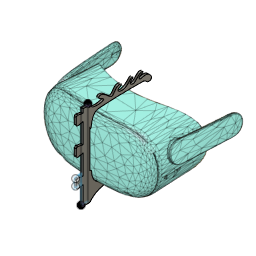
Quest Flat Holder To Store v1 (Autodesk Fusion 360 design; units mm, degrees)
Autodesk Fusion 360 part; units mm, degrees
other "Fonction de maillage de base1"
other "Modifier1"
sketch "Esquisse2" plane through (0, 0, 0) normal (1, 0, 0) x (0, 1, 0)
  line L0 (0, 0) -> (85, 0) construction
  line L1 (85, 0) -> (85, -20) construction
  line L2 (85, -20) -> (0, -20) construction
  line L3 (0, -20) -> (0, 0) construction
  spline S0 degree 5 poles (0, 20) (0.1728, 20.096) (0.5018, 20.2595) (0.9458, 20.4196) (1.4388, 20.4623) (1.8937, 20.2348) (2.1997, 19.7392) (2.3839, 19.0043) (2.486, 18.0734) (2.5511, 16.9974) (2.6227, 15.8294) (2.7376, 14.6194) (2.9173, 13.4073) (3.1676, 12.2219) (3.4842, 11.0828) (3.8558, 10.002) (4.2682, 8.9856) (4.7086, 8.0352) (5.1695, 7.1497) (5.6506, 6.3263) (6.1549, 5.5614) (6.688, 4.851) (7.2552, 4.1918) (7.8594, 3.582) (8.5004, 3.0212) (9.177, 2.5098) (9.8879, 2.0486) (10.6332, 1.6379) (11.416, 1.2771) (12.2414, 0.9646) (13.1157, 0.6985) (14.0453, 0.4767) (15.0358, 0.297) (16.0906, 0.1581) (17.2121, 0.0586) (18.4011, -0.0021) (19.4067, -0.0202) (20.1915, -0.0167) (20.7282, -0.0068) (21, 0) knots 0 0 0 0 0 0 0.028571 0.057143 0.085714 0.114286 0.142857 0.171429 0.2 0.228571 0.257143 0.285714 0.314286 0.342857 0.371429 0.4 0.428571 0.457143 0.485714 0.514286 0.542857 0.571429 0.6 0.628571 0.657143 0.685714 0.714286 0.742857 0.771429 0.8 0.828571 0.857143 0.885714 0.914286 0.942857 0.971429 1 1 1 1 1 1
  spline S1 degree 5 poles (0, -20) (0.5064, -19.2983) (1.5674, -17.9422) (3.3034, -16.0502) (5.9091, -13.8142) (9.6604, -11.5007) (13.9117, -9.6603) (18.656, -8.2562) (23.8646, -7.2118) (29.4972, -6.4287) (35.5074, -5.8004) (41.8485, -5.2261) (48.4776, -4.6251) (55.3593, -3.9458) (62.4652, -3.1575) (69.7745, -2.245) (75.7737, -1.4114) (80.3552, -0.7281) (83.4457, -0.247) (85, 0) knots 0 0 0 0 0 0 0.066667 0.133333 0.2 0.266667 0.333333 0.4 0.466667 0.533333 0.6 0.666667 0.733333 0.8 0.866667 0.933333 1 1 1 1 1 1
  spline S2 degree 5 poles (85, 0) (85.575, 0.0875) (86.7285, 0.3082) (88.4686, 0.7768) (90.8086, 1.677) (93.7558, 3.2561) (96.6909, 5.2678) (99.5457, 7.6663) (102.2047, 10.3705) (104.4963, 13.2564) (106.1711, 16.1422) (106.9676, 18.8127) (106.7051, 21.0543) (105.3645, 22.6857) (103.1826, 23.5917) (100.722, 23.753) (98.6234, 23.2199) (97.4016, 22.0921) (97.1788, 20.4954) (97.593, 18.5638) (98.0858, 16.4294) (98.097, 14.2122) (97.3281, 12.0076) (95.7145, 9.8887) (93.3441, 7.9095) (90.3947, 6.1092) (87.0665, 4.5151) (83.512, 3.1458) (79.8386, 2.0134) (76.1175, 1.1247) (72.3914, 0.4826) (69.4234, 0.1665) (67.2077, 0.0403) (65.7351, 0.0052) (65, 0) knots 0 0 0 0 0 0 0.033333 0.066667 0.1 0.133333 0.166667 0.2 0.233333 0.266667 0.3 0.333333 0.366667 0.4 0.433333 0.466667 0.5 0.533333 0.566667 0.6 0.633333 0.666667 0.7 0.733333 0.766667 0.8 0.833333 0.866667 0.9 0.933333 0.966667 1 1 1 1 1 1
  line L4 (0, 0) -> (0, 20)
  line L5 (21, 0) -> (65, 0)
  line L6 (0, 0) -> (0, -20)
  point P0 (2, 20)
  point P1 (2.6822, 15.27)
  point P2 (4.5, 8.5)
  point P3 (7, 4.5)
  point P4 (10, 2)
  point P5 (14, 0.5)
  point P6 (13.4129, -10)
  point P7 (40.3283, -5.3657)
  point P8 (102.6529, 11.0428)
  point P9 (105.3058, 22.3913)
  point P10 (97.9366, 22.3913)
  point P11 (98, 16)
  point P12 (90, 6)
  dimension "d3" = 85
  dimension "d4" = 20
  constraint horizontal L0
  constraint vertical L1
  constraint horizontal L2
  constraint vertical L3
  constraint coincident L0.start L3.end
  constraint coincident L0 S0.end
  constraint coincident L0 S2.end
  constraint perpendicular L0 L4
  measures "d3" distance of L0.start L0.end
  measures "d4" distance of L0.start L2.end
extrude "Extrusion1" add sketch "Esquisse2" along normal blind 3 makes body 1
sketch "Esquisse3" plane through (0, 0, 0) normal (1, 0, 0) x (0, 1, 0)
  line L0 (0, 94.6179) -> (85, 94.6179) construction
  line L1 (85, 94.6179) -> (85, 114.6179) construction
  line L2 (85, 114.6179) -> (0, 114.6179) construction
  line L3 (0, 114.6179) -> (0, 94.6179) construction
  line L4 (0, 94.6179) -> (0, 75)
  spline S0 degree 5 poles (2, 75) (2.0202, 75.3852) (2.0715, 76.1534) (2.1807, 77.2986) (2.3912, 78.8117) (2.7621, 80.6771) (3.2396, 82.5084) (3.8209, 84.2894) (4.5015, 85.9934) (5.2735, 87.579) (6.1296, 88.9972) (7.0689, 90.2031) (8.1023, 91.166) (9.258, 91.8812) (10.5862, 92.3785) (12.1486, 92.7086) (14.0103, 92.9314) (16.2308, 93.1038) (18.8544, 93.2665) (21.9061, 93.4406) (25.3926, 93.633) (29.3013, 93.8393) (33.6009, 94.0477) (38.24, 94.2424) (43.1479, 94.4068) (48.2328, 94.5281) (53.3833, 94.5985) (58.4639, 94.6234) (63.3238, 94.6152) (67.7739, 94.6186) (71.6525, 94.6526) (74.8757, 94.68) (77.4148, 94.6435) (79.3006, 94.4768) (80.6174, 94.1256) (81.5018, 93.5651) (82.137, 92.8177) (82.7573, 91.9753) (83.5789, 91.1727) (84.729, 90.5551) (86.1523, 90.2442) (87.6474, 90.3207) (88.9663, 90.8167) (89.8915, 91.7056) (90.3307, 92.8885) (90.2941, 94.2263) (89.8594, 95.5735) (89.1393, 96.8178) (88.2552, 97.8964) (87.3226, 98.7772) (86.4355, 99.4496) (85.8043, 99.8181) (85.3821, 99.9986) (85.1236, 100.0764) (85, 100.1046) knots 0 0 0 0 0 0 0.02 0.04 0.06 0.08 0.1 0.12 0.14 0.16 0.18 0.2 0.22 0.24 0.26 0.28 0.3 0.32 0.34 0.36 0.38 0.4 0.42 0.44 0.46 0.48 0.5 0.52 0.54 0.56 0.58 0.6 0.62 0.64 0.66 0.68 0.7 0.72 0.74 0.76 0.78 0.8 0.82 0.84 0.86 0.88 0.9 0.92 0.94 0.96 0.98 1 1 1 1 1 1
  line L5 (50.046, 94.6179) -> (76, 94.6179)
  spline S1 degree 5 poles (0, 75) (0.04, 74.8483) (0.12, 74.5582) (0.24, 74.1627) (0.4, 73.7162) (0.6, 73.3019) (0.8, 73.0442) (1, 72.956) (1.2, 73.0442) (1.4, 73.3019) (1.6, 73.7162) (1.76, 74.1627) (1.88, 74.5582) (1.96, 74.8483) (2, 75) knots 0 0 0 0 0 0 0.1 0.2 0.3 0.4 0.5 0.6 0.7 0.8 0.9 1 1 1 1 1 1
  line L6 (0, 94.6179) -> (0, 110)
  spline S2 degree 5 poles (0, 103.8612) (0.0594, 103.6458) (0.2491, 103.0393) (0.6491, 102.1073) (1.4026, 100.9699) (2.7032, 99.7974) (4.5145, 98.8515) (6.6398, 98.2367) (8.9921, 97.9297) (11.4551, 97.8986) (13.8795, 98.1029) (16.1006, 98.4961) (17.9568, 99.0296) (19.3078, 99.6559) (20.0524, 100.3325) (20.147, 101.025) (19.6236, 101.7106) (18.6074, 102.3817) (17.2834, 103.0411) (15.8653, 103.6979) (14.5626, 104.3634) (13.5514, 105.0463) (12.9359, 105.749) (12.7503, 106.4616) (12.9835, 107.155) (13.5974, 107.7726) (14.5449, 108.2285) (15.7707, 108.4296) (17.2154, 108.2956) (18.8182, 107.7781) (20.5203, 106.8841) (22.2667, 105.6788) (24.0079, 104.2665) (25.7004, 102.7783) (27.3086, 101.3566) (28.8054, 100.1412) (30.1742, 99.2545) (31.4094, 98.7879) (32.5181, 98.7853) (33.5207, 99.2355) (34.4477, 100.085) (35.3379, 101.2458) (36.2356, 102.6055) (37.1892, 104.0369) (38.2469, 105.4075) (39.4424, 106.5917) (40.782, 107.4827) (42.2327, 108.0039) (43.7068, 108.122) (45.054, 107.8564) (46.0348, 107.2969) (46.4036, 106.5721) (46.0116, 105.8057) (44.9262, 105.07) (43.4777, 104.3604) (42.1029, 103.6356) (41.1858, 102.8524) (40.98, 101.9881) (41.3072, 101.1045) (41.8959, 100.2884) (42.7, 99.5867) (43.7084, 99.0408) (44.9511, 98.6814) (46.4159, 98.543) (48.0582, 98.6571) (49.8113, 99.0469) (51.5976, 99.7212) (53.3396, 100.6684) (54.9707, 101.8501) (56.4453, 103.1961) (57.753, 104.5956) (58.9108, 105.9106) (59.9459, 107.0023) (60.8814, 107.752) (61.7197, 108.0872) (62.4307, 107.9988) (62.9269, 107.5773) (63.0956, 106.978) (62.8745, 106.3345) (62.3108, 105.6926) (61.5214, 105.0471) (60.6581, 104.3739) (59.8672, 103.6713) (59.2651, 102.9698) (58.9433, 102.2883) (58.9681, 101.5986) (59.3795, 100.7877) (60.1369, 99.9443) (61.1612, 99.226) (62.3546, 98.8155) (63.6313, 98.8337) (64.9349, 99.3) (66.2302, 100.1631) (67.5002, 101.3194) (68.7406, 102.6368) (69.9563, 103.9754) (71.156, 105.2098) (72.3483, 106.2513) (73.5347, 107.045) (74.7026, 107.5654) (75.8178, 107.8129) (76.8197, 107.8097) (77.6089, 107.5967) (78.0566, 107.227) (78.0583, 106.7528) (77.5908, 106.211) (76.7239, 105.6208) (75.589, 104.9939) (74.3615, 104.3412) (73.2363, 103.681) (72.4025, 103.0412) (71.97, 102.424) (71.9613, 101.8181) (72.1553, 101.104) (72.4975, 100.3787) (73.0531, 99.8457) (73.89, 99.6554) (75.0119, 99.7998) (76.3766, 100.1751) (77.9071, 100.6231) (79.5054, 100.9824) (81.0644, 101.1308) (82.4822, 101.0442) (83.6696, 100.7811) (84.378, 100.5037) (84.7522, 100.2982) (84.9294, 100.168) (85, 100.1046) knots 0.01975659 0.01975659 0.01975659 0.01975659 0.01975659 0.01975659 0.024 0.032 0.04 0.048 0.056 0.064 0.072 0.08 0.088 0.096 0.104 0.112 0.12 0.128 0.136 0.144 0.152 0.16 0.168 0.176 0.184 0.192 0.2 0.208 0.216 0.224 0.232 0.24 0.248 0.256 0.264 0.272 0.28 0.288 0.296 0.304 0.312 0.32 0.328 0.336 0.344 0.352 0.36 0.368 0.376 0.384 0.392 0.4 0.408 0.416 0.424 0.432 0.44 0.448 0.456 0.464 0.472 0.48 0.488 0.496 0.504 0.512 0.52 0.528 0.536 0.544 0.552 0.56 0.568 0.576 0.584 0.592 0.6 0.608 0.616 0.624 0.632 0.64 0.648 0.656 0.664 0.672 0.68 0.688 0.696 0.704 0.712 0.72 0.728 0.736 0.744 0.752 0.76 0.768 0.776 0.784 0.792 0.8 0.808 0.816 0.824 0.832 0.84 0.848 0.856 0.864 0.872 0.88 0.888 0.896 0.904 0.912 0.92 0.928 0.936 0.944 0.952 0.96 0.968 0.976 0.984 0.992 1 1 1 1 1 1
  line L7 (-2.2438, 111.9912) -> (2.2438, 95.7313)
  line L8 (41.0002, 107.9903) -> (41.2219, 96.0623)
  line L9 (59, 107.9346) -> (59, 96.0654)
  line L10 (72, 108.1104) -> (72, 95.8896)
  line L11 (82.3506, 102.4836) -> (87.6494, 97.7257)
  point P0 (4.0472, 84.8089)
  point P1 (8, 91)
  point P2 (15, 93)
  point P3 (63.023, 94.6179)
  point P4 (81.5564, 93.4173)
  point P5 (84, 91)
  point P6 (89, 91)
  point P7 (90, 95)
  point P8 (87, 99)
  point P9 (1, 73)
  point P10 (9, 98)
  point P11 (20, 101)
  point P12 (14.2323, 104.6179)
  point P13 (13, 107)
  point P14 (18, 108)
  point P15 (31, 99)
  point P16 (36.0384, 102.3089)
  point P17 (44, 108)
  point P18 (46, 106)
  point P19 (41.111, 102.0263)
  point P20 (44, 99)
  point P21 (55.43, 102.3089)
  point P22 (62, 108)
  point P23 (63, 107)
  point P24 (60.9799, 104.6179)
  point P25 (59, 102)
  point P26 (62, 99)
  point P27 (70, 104)
  point P28 (76.5063, 107.7784)
  point P29 (78, 107)
  point P30 (74.8889, 104.6179)
  point P31 (72, 102)
  point P32 (73, 100)
  point P33 (80, 101)
  dimension "d7" = 85
  dimension "d8" = 20
  constraint horizontal L0
  constraint vertical L1
  constraint horizontal L2
  constraint vertical L3
  constraint perpendicular L0 L4
  constraint coincident L0 P3
  constraint coincident L1 S0.end
  constraint midpoint P3 L5
  constraint coincident L0 L5.end
  constraint coincident L3 L6.end
  constraint coincident L3 S2.start
  constraint midpoint S2.start L7
  constraint midpoint P19 L8
  constraint midpoint P25 L9
  constraint midpoint P31 L10
  constraint midpoint S0.end L11
  measures "d7" distance of L0.start L0.end
  measures "d8" distance of L0.start L2.end
sketch "Esquisse4" plane through (0, 0, 0) normal (1, 0, 0) x (0, 1, 0)
  line L0 (0, 103.8612) -> (-10, 103.8612)
  line L1 (-10, 103.8612) -> (-10, -20)
  line L2 (-10, -20) -> (0, -20)
  line L3 (0, -20) -> (0, 103.8612)
  point P0 (0, 103.8612)
  dimension "d11" = 10
  constraint horizontal L0
  constraint vertical L1
  constraint horizontal L2
  constraint vertical L3
  constraint coincident P0 L0.start
  measures "d11" distance of P0 L0.end
extrude "Extrusion2" add sketch "Esquisse3" sketch "Esquisse4" along normal blind 3 contours L4 S0 S1 L6 S2 L8 L9 L10 | S2 L8 | S2 L9 | S2 L10 of sketch 2 bodies 1
sketch "Esquisse5" plane through (0, 0, 0) normal (1, 0, 0) x (0, 1, 0)
  line L0 (-10, -20) -> (-10, 20)
  line L1 (-10, 20) -> (-20, 20)
  line L2 (-20, 17.5851) -> (-20, 7.9635)
  line L3 (-20, 5.5) -> (-10, 5.5)
  line L4 (-10, 5.5) -> (-10, 20)
  line L5 (-17.6274, 19.5501) -> (-10, 18.1039)
  line L6 (-17.5891, 6.0061) -> (-10, 7.5994)
  arc A0 (-17.6274, 19.5501) -> (-20, 17.5851) centre (-18, 17.5851) ccw
  arc A1 (-20, 7.9635) -> (-17.5891, 6.0061) centre (-18, 7.9635) ccw
  point P0 (-10, -20)
  dimension "d12" = 40
  dimension "d13" = 10
  dimension "d14" = 14.5
  dimension "d15" = 2
  dimension "d16" = 2
  constraint coincident P0 L0.start
  constraint horizontal L1
  constraint vertical L2
  constraint horizontal L3
  constraint vertical L4
  constraint coincident L0 L5.end
  constraint coincident L4 L5.end
  constraint coincident L4 L6.end
  constraint coincident L1.end L2
  constraint coincident L1.end L5
  constraint tangent L2 A0
  constraint tangent L5 A0
  constraint coincident L3.start L6
  constraint coincident L3.start L2
  constraint tangent L6 A1
  constraint tangent L2 A1
  measures "d12" distance of P0 L0.end
  measures "d13" distance of L0.end L1.end
  measures "d14" distance of L0.end L3.end
  measures "d15" radius of A0
  measures "d16" radius of A1
extrude "Extrusion3" add sketch "Esquisse5" along normal blind 3 separate body makes body 2
pattern_linear "Réseau R1" count 3 spacing 40 along (0, 0, 1) of bodies 2 makes body 3 at (0, -13.3333, 54.4295) makes body 4 at (0, -13.3333, 94.4295)
combine "Combiner1" operation add target body 4 tool bodies 1 3 2
